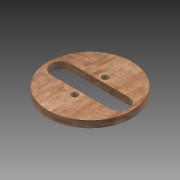
# Autodesk Inventor part: 1
Saved by Autodesk Inventor 2015 (Build 190159000, 159)
## iProperties
Created: 2016-01-31
Part Number: 1
Material: Generic
Document SubType Name: Modeling
Designer: david
Density: 1 g/cm^3
Appearance: Birch - Natural Polished
Mass: 3.97957 g
Surface Area: 31.1882 cm^2
Volume: 3.97957 cm^3
Author: david
Autodesk Inventor part; units mm, degrees
ref_plane "YZ Plane" through (0, 0, 0) normal (1, 0, 0) x (0, 1, 0)
ref_plane "XZ Plane" through (0, 0, 0) normal (0, 1, 0) x (-1, 0, 0)
ref_plane "XY Plane" through (0, 0, 0) normal (0, 0, 1) x (1, 0, 0)
sketch "Sketch1" plane through (0, 0, 0) normal (0, 0, 1) x (1, 0, 0)
  circle A0 centre (0, 0) radius 22
  dimension "d0" = 44
  constraints: 1 centre point, 1 coincident
  measures "d0" diameter of A0
extrude "Extrusion1" add sketch "Sketch1" along normal blind 3.6
sketch "Sketch2" plane through (0, 0, 3.6) normal (0, 0, 1) x (1, 0, 0)
  line L0 (15.3, 0) -> (-15.3, 0) construction
  line L1 (15.3, 5.15) -> (-15.3, 5.15)
  line L2 (-15.3, -5.15) -> (15.3, -5.15)
  arc A0 (15.3, -5.15) -> (15.3, 5.15) centre (15.3, 0) ccw
  arc A1 (-15.3, 5.15) -> (-15.3, -5.15) centre (-15.3, 0) ccw
  point P0 (0, 0)
  dimension "d3" = 15.3
  dimension "d4" = 10.3
  constraints: 8 end point, 4 point on circle, 4 tangent, 2 centre point, 1 horizontal, 1 midpoint, 1 parallel
  measures "d3" distance of point (0, 0) L0.end
  measures "d4" diameter of A1
extrude "Extrusion2" cut sketch "Sketch2" against normal blind 3.6
sketch "Sketch3" plane through (0, 0, 3.6) normal (0, 0, 1) x (1, 0, 0)
  line L0 (-2.6, 9.8) -> (2.6, 9.8)
  line L1 (2.6, 9.8) -> (2.6, 6)
  line L2 (2.6, 6) -> (-2.6, 6)
  line L3 (-2.6, 6) -> (-2.6, 9.8)
  line L4 (-2.6, 9.8) -> (2.6, 6) construction
  line L5 (2.6, 9.8) -> (-2.6, 6) construction
  line L6 (-30.8, 0) -> (30.8, 0) projected
  line L7 (-30.8, 0) -> (30.8, 0) projected
  line L8 (-2.6, -9.8) -> (2.6, -9.8)
  line L9 (2.6, -9.8) -> (2.6, -6)
  line L10 (2.6, -6) -> (-2.6, -6)
  line L11 (-2.6, -6) -> (-2.6, -9.8)
  line L12 (-2.6, -9.8) -> (2.6, -6) construction
  line L13 (2.6, -9.8) -> (-2.6, -6) construction
  circle A0 centre (0, -7.9) radius 1.625
  circle A1 centre (0, 7.9) radius 1.625
  point P0 (0, 0)
  dimension "d7" = 5.2
  dimension "d8" = 3.8
  dimension "d9" = 6
  dimension "d10" = 6
  dimension "d13" = 0
  dimension "d14" = 3.25
  dimension "d15" = 3.25
  constraints: 24 end point, 5 symmetric about line, 4 midpoint, 2 centre point, 2 coincident, 2 parallel, 1 horizontal, 1 perpendicular
  measures "d7" distance of L1.end L2.end
  measures "d8" distance of L0.end L1.end
  measures "d9" distance from line of L2.end L6
  measures "d10" distance from line of L6 L1.end
  measures "d13" horizontal distance of point (0, 0) point (0, 7.9)
  measures "d14" diameter of A0
  measures "d15" diameter of A1
extrude "Extrusion3" cut sketch "Sketch3" against normal blind 10 contours A0 | A1
body "Solid1"
